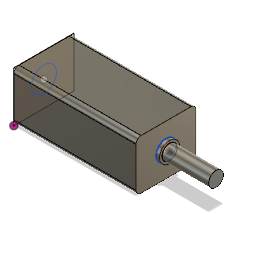
morter v2 (Autodesk Fusion 360 design; units mm, degrees)
Autodesk Fusion 360 part; units mm, degrees
sketch "スケッチ1" plane through (0, 0, 0) normal (1, 0, 0) x (0, 0, -1)
  line L0 (0, 0) -> (12, 0)
  line L1 (12, 0) -> (12, 10)
  line L2 (12, 10) -> (0, 10)
  line L3 (0, 10) -> (0, 0)
  dimension "d1" = 10
  dimension "d2" = 12
  measures "d2" distance of L0.start
extrude "押し出し1" add sketch "スケッチ1" along normal blind 24.4 makes body 1
fillet "フィレット1" radius 1 1 edges at (12.2, 10, -12) on bodies 1
fillet "フィレット2" radius 1 1 edges at (12.2, 10, 0) on bodies 1
fillet "フィレット3" radius 1 1 edges at (12.2, 0, -12) on bodies 1
fillet "フィレット4" radius 1 1 edges at (12.2, 0, 0) on bodies 1
sketch "スケッチ2" plane through (24.4, 0, 0) normal (1, 0, 0) x (0, 0, -1)
  arc A0 (0, 1) -> (1, 0) centre (1, 1) ccw
  line L0 (1, 0) -> (11, 0)
  arc A1 (11, 0) -> (12, 1) centre (11, 1) ccw
  line L1 (12, 1) -> (12, 9)
  arc A2 (12, 9) -> (11, 10) centre (11, 9) ccw
  line L2 (11, 10) -> (1, 10)
  arc A3 (1, 10) -> (0, 9) centre (1, 9) ccw
  line L3 (0, 9) -> (0, 1)
  circle A4 centre (6, 5) radius 2
  dimension "d18" = 2
  measures "d18" radius of A4
extrude "押し出し2" add sketch "スケッチ2" along normal blind 0.7 contours A4 bodies 1
sketch "スケッチ3" plane through (25.1, 0, 0) normal (1, 0, 0) x (0, 0, -1)
  circle A0 centre (6, 5) radius 2
  circle A1 centre (6, 5) radius 1.5
  dimension "d12" = 3
  measures "d12" diameter of A1
extrude "押し出し3" add sketch "スケッチ3" along normal blind 9.3 contours A1 bodies 1
sketch "スケッチ4" plane through (0, 0, 0) normal (-1, 0, 0) x (0, 0, 1)
  arc A0 (-1, 0) -> (0, 1) centre (-1, 1) ccw
  line L0 (0, 1) -> (0, 9)
  arc A1 (0, 9) -> (-1, 10) centre (-1, 9) ccw
  line L1 (-1, 10) -> (-11, 10)
  arc A2 (-11, 10) -> (-12, 9) centre (-11, 9) ccw
  line L2 (-12, 9) -> (-12, 1)
  arc A3 (-12, 1) -> (-11, 0) centre (-11, 1) ccw
  line L3 (-11, 0) -> (-1, 0)
  circle A4 centre (-6, 5) radius 2.5
  dimension "d15" = 5
  measures "d15" diameter of A4
extrude "押し出し1'" add sketch "スケッチ4" along normal blind 0.8 separate body contours A4 makes body 2 in component "Component"
component "Component" placed x (1, 0, 0) y (0, 1, 0) z (0, 0, 1) at (0, 0, 0)
